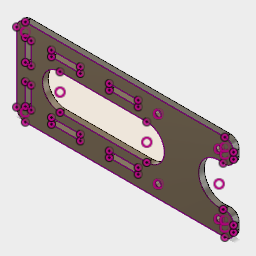
Lower (Autodesk Fusion 360 design; units mm, degrees)
Autodesk Fusion 360 part; units mm, degrees
sketch "Sketch1" plane through (0, 0, -20.5) normal (0, 0, -1) x (-1, 0, 0)
  line L0 (-5, 0) -> (-5, -15)
  line L1 (-5, -15) -> (70, -15)
  line L2 (70, -15) -> (70, 0)
  circle A0 centre (0, -10.5) radius 1
  circle A1 centre (21, -10.5) radius 1
  circle A2 centre (0, 0) radius 7.0711
  line L3 (67, -10.3624) -> (65, -10.3624)
  line L4 (65, -10.3624) -> (65, -2.8871)
  line L5 (65, -2.8871) -> (67, -2.8871)
  line L6 (67, -2.8871) -> (67, -10.3624)
  line L7 (100, 0) -> (42, 0) construction
  line L8 (-5, 15) -> (70, 15)
  line L9 (70, 15) -> (70, 0)
  line L10 (67, 10.3624) -> (65, 10.3624)
  line L11 (67, 2.8871) -> (67, 10.3624)
  line L12 (65, 10.3624) -> (65, 2.8871)
  line L13 (65, 2.8871) -> (67, 2.8871)
  circle A3 centre (21, 10.5) radius 1
  circle A4 centre (0, 10.5) radius 1
  line L14 (-5, 0) -> (-5, 15)
  line L15 (27.9727, 11.0949) -> (37.9727, 11.0949)
  line L16 (37.9727, 11.0949) -> (37.9727, 9.0949)
  line L17 (37.9727, 9.0949) -> (27.9727, 9.0949)
  line L18 (27.9727, 9.0949) -> (27.9727, 11.0949)
  line L19 (42.9727, 11.2127) -> (42.9727, -12.2873) construction
  line L20 (42.9727, -11.2127) -> (42.9727, 12.2873) construction
  line L21 (37.9727, -11.0949) -> (37.9727, -9.0949)
  line L22 (37.9727, -9.0949) -> (27.9727, -9.0949)
  line L23 (27.9727, -9.0949) -> (27.9727, -11.0949)
  line L24 (27.9727, -11.0949) -> (37.9727, -11.0949)
  line L25 (57.9727, 11.0949) -> (47.9727, 11.0949)
  line L26 (47.9727, 11.0949) -> (47.9727, 9.0949)
  line L27 (47.9727, 9.0949) -> (57.9727, 9.0949)
  line L28 (57.9727, 9.0949) -> (57.9727, 11.0949)
  line L29 (47.9727, -11.0949) -> (47.9727, -9.0949)
  line L30 (57.9727, -9.0949) -> (57.9727, -11.0949)
  line L31 (47.9727, -9.0949) -> (57.9727, -9.0949)
  line L32 (57.9727, -11.0949) -> (47.9727, -11.0949)
  dimension "d1" = 75
  dimension "d3" = 2
  dimension "d4" = 3
  dimension "d77" = 0
  dimension "d78" = 0
  dimension "d79" = 0
  dimension "d80" = 0
  dimension "d93" = 10
  dimension "d94" = 2
  dimension "d95" = 10
  measures "d1" distance of L0.end L1.end
  measures "d3" distance of L4 L6
  measures "d4" distance of L2 L6
  measures "d93" distance of L15.start L15.end
  measures "d94" distance of L15.start L17.end
  measures "d95" distance of L16 L26
extrude "Extrude1" add sketch "Sketch1" along normal blind 2 contours L0 L1 L2 A2 L8 L9 L14
sketch "Sketch2" plane through (0, 0, -22.5) normal (0, 0, -1) x (-1, 0, 0)
  line L0 (25, -6.0704) -> (55, -6.0704)
  arc A0 (55, -6.0704) -> (55, 6.0704) centre (55, 0) ccw
  line L1 (55, 6.0704) -> (25, 6.0704)
  arc A1 (25, 6.0704) -> (25, -6.0704) centre (25, 0) ccw
  line L2 (25, 0) -> (55, 0) construction
  line L3 (100, 0) -> (42, 0)
extrude "Extrude2" cut sketch "Sketch2" against normal blind 2
fillet "Fillet1" radius 3 6 edges at (5, 15, -21.5) (5, 5, -21.5) (5, -5, -21.5) (5, -15, -21.5) (-70, 15, -21.5) (-70, -15, -21.5)
sketch "Sketch3" plane through (0, 0, -20.5) normal (0, 0, 1) x (1, 0, 0)
sketch "projection" plane through (0, 0, -20.5) normal (0, 0, 1) x (1, 0, 0)
  line L0 (-25, -6.0704) -> (-55, -6.0704)
  arc A0 (-55, 6.0704) -> (-55, -6.0704) centre (-55, 0) ccw
  line L1 (-55, 6.0704) -> (-25, 6.0704)
  arc A1 (-25, -6.0704) -> (-25, 6.0704) centre (-25, 0) ccw
  circle A2 centre (-21, 10.5) radius 1
  line L2 (-57.9727, -11.0949) -> (-57.9727, -9.0949)
  line L3 (-57.9727, -9.0949) -> (-47.9727, -9.0949)
  line L4 (-47.9727, -9.0949) -> (-47.9727, -11.0949)
  line L5 (-47.9727, -11.0949) -> (-57.9727, -11.0949)
  circle A3 centre (0, 10.5) radius 1
  line L6 (-65, 2.8871) -> (-67, 2.8871)
  line L7 (-67, 2.8871) -> (-67, 10.3624)
  line L8 (-67, 10.3624) -> (-65, 10.3624)
  line L9 (-65, 10.3624) -> (-65, 2.8871)
  line L10 (-27.9727, -11.0949) -> (-37.9727, -11.0949)
  line L11 (-37.9727, -11.0949) -> (-37.9727, -9.0949)
  line L12 (-37.9727, -9.0949) -> (-27.9727, -9.0949)
  line L13 (-27.9727, -9.0949) -> (-27.9727, -11.0949)
  circle A4 centre (0, -10.5) radius 1
  line L14 (-57.9727, 9.0949) -> (-57.9727, 11.0949)
  line L15 (-57.9727, 11.0949) -> (-47.9727, 11.0949)
  line L16 (-47.9727, 11.0949) -> (-47.9727, 9.0949)
  line L17 (-47.9727, 9.0949) -> (-57.9727, 9.0949)
  circle A5 centre (-21, -10.5) radius 1
  line L18 (-67, -2.8871) -> (-65, -2.8871)
  line L19 (-65, -2.8871) -> (-65, -10.3624)
  line L20 (-65, -10.3624) -> (-67, -10.3624)
  line L21 (-67, -10.3624) -> (-67, -2.8871)
  line L22 (-27.9727, 9.0949) -> (-37.9727, 9.0949)
  line L23 (-37.9727, 9.0949) -> (-37.9727, 11.0949)
  line L24 (-37.9727, 11.0949) -> (-27.9727, 11.0949)
  line L25 (-27.9727, 11.0949) -> (-27.9727, 9.0949)
  arc A6 (-70, -12) -> (-67, -15) centre (-67, -12) ccw
  line L26 (-67, -15) -> (2, -15)
  arc A7 (2, -15) -> (5, -12) centre (2, -12) ccw
  line L27 (5, -12) -> (5, -9.8705)
  arc A8 (5, -9.8705) -> (1.4042, -6.9302) centre (2, -9.8705) ccw
  arc A9 (1.4042, 6.9302) -> (1.4042, -6.9302) centre (0, 0) ccw
  arc A10 (1.4042, 6.9302) -> (5, 9.8705) centre (2, 9.8705) ccw
  line L28 (5, 9.8705) -> (5, 12)
  arc A11 (5, 12) -> (2, 15) centre (2, 12) ccw
  line L29 (2, 15) -> (-67, 15)
  arc A12 (-67, 15) -> (-70, 12) centre (-67, 12) ccw
  line L30 (-70, 12) -> (-70, -12)
equation "thiccness = 2 mm"
equation "d3 = thiccness"
equation "d11 = thiccness"
equation "d94 = thiccness"
equation "d96 = -thiccness"
named bodies: "leg"
